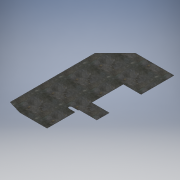
# Autodesk Inventor part: Gearbox-Side Cover Part 1
Saved by Autodesk Inventor 2018 (Build 220112000, 112)
## iProperties
Created: 2018-08-07
Part Number: Gearbox-Side Cover Part 1
Material: Steel
Document SubType Name: Modeling
Designer: P301319
Density: 7.85 g/cm^3
Appearance: Plate
Author: P301319
Autodesk Inventor part; units mm, degrees
ref_plane "YZ Plane" through (0, 0, 0) normal (1, 0, 0) x (0, 1, 0)
ref_plane "XZ Plane" through (0, 0, 0) normal (0, 1, 0) x (-1, 0, 0)
ref_plane "XY Plane" through (0, 0, 0) normal (0, 0, 1) x (1, 0, 0)
sketch "Sketch1" plane through (0, 0, 0) normal (0, 0, 1) x (1, 0, 0)
  line L0 (0, 0) -> (200, 0)
  line L1 (0, 0) -> (-100, 30)
  line L2 (0, 0) -> (236.9147, 0) construction
  line L3 (-100, 650) -> (-100, 30)
  line L4 (-100, 650) -> (50, 800)
  line L5 (50, 800) -> (330, 800)
  line L6 (330, 800) -> (330, 560)
  line L7 (330, 560) -> (200, 560)
  line L8 (200, 235) -> (330, 235)
  line L9 (330, 325) -> (330, 235)
  line L10 (155, 203.5) -> (200, 203.5)
  line L11 (155, 228.5) -> (200, 228.5)
  arc A0 (155, 228.5) -> (155, 203.5) centre (155, 216) ccw
  line L12 (200, 0) -> (200, 203.5)
  line L13 (200, 228.5) -> (200, 235)
  line L14 (200, 560) -> (200, 325)
  line L15 (200, 325) -> (330, 325)
  dimension "d0" = 200
  dimension "d3" = 100
  dimension "d6" = 800
  dimension "d7" = 240
  dimension "d8" = 130
  dimension "d11" = 235
  dimension "d14" = 25
  dimension "d16" = 216
  dimension "d18" = 45
  dimension "d19" = 430
  dimension "d20" = 135
  dimension "d22" = 130
  dimension "d23" = 235
  dimension "d24" = 280
  dimension "d25" = 30
  constraints: 34 end point, 6 horizontal, 4 perpendicular, 4 vertical, 2 point on circle, 2 tangent, 1 centre point, 1 parallel, 1 vertical alignment
  measures "d0" distance of L0.start L0.end
  measures "d3" distance from line of L0.start L3
  measures "d6" distance between parallel lines of L0 L5
  measures "d7" distance of L5.end L6.end
  measures "d8" distance of L6.end L7.end
  measures "d11" distance of L0.end L8.start
  measures "d14" distance between parallel lines of L10 L11
  measures "d16" vertical distance of L0.start A0.centre
  measures "d18" distance of L10.start L10.end
  measures "d19" distance between parallel lines of L3 L6
  measures "d20" angle of L5 L4
  measures "d22" distance of L14.end L9.start
  measures "d23" distance of L7.end L14.end
  measures "d24" distance of L4.end L5.end
  measures "d25" vertical distance of L0.start L1.end
extrude "Extrusion1" add sketch "Sketch1" along normal blind 1.6
equation "\"d22\" = d8"
equation "\"BendRadius\" = Thickness"
equation "\"BendReliefWidth\" = Thickness"
equation "\"BendReliefDepth\" = 0.5 * Thickness"
equation "\"CornerReliefSize\" = 4 * Thickness"
equation "\"MinimumRemnant\" = 2 * Thickness"
equation "\"TransitionRadius\" = BendRadius"
equation "\"JacobiRadiusSize\" = Thickness"
equation "\"GapSize\" = Thickness"
equation "\"Thickness\" = 0.5"
body "Solid1"
